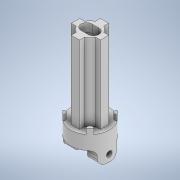
# Autodesk Inventor part: upper plug
Saved by Autodesk Inventor 2022 (Build 260153000, 153)
## iProperties
Created: 2022-03-20
Part Number: upper plug
Material: Generic
Document SubType Name: Modeling
Designer: Dahway
Density: 1 g/cm^3
Appearance: Default
Author: Dahway
Autodesk Inventor part; units mm, degrees
ref_plane "YZ Plane" through (0, 0, 0) normal (1, 0, 0) x (0, 1, 0)
ref_plane "XZ Plane" through (0, 0, 0) normal (0, 1, 0) x (-1, 0, 0)
ref_plane "XY Plane" through (0, 0, 0) normal (0, 0, 1) x (1, 0, 0)
sketch "Sketch1" plane through (0, 0, 0) normal (0, 1, 0) x (-1, 0, 0)
  circle A0 centre (0, 0) radius 7
  dimension "d0" = 14
  constraints: 1 centre point, 1 coincident
  measures "d0" diameter of A0
extrude "Extrusion1" add sketch "Sketch1" along normal blind 5
sketch "Sketch2" plane through (0, 5, 0) normal (0, 1, 0) x (1, 0, 0)
  circle A0 centre (0, 0) radius 3.75
  line L0 (-5.25, -1.5) -> (-2.25, -1.5)
  line L1 (-2.25, -1.5) -> (-2.25, 1.5)
  line L2 (-2.25, 1.5) -> (-5.25, 1.5)
  line L3 (-5.25, 1.5) -> (-5.25, -1.5)
  line L4 (-5.25, -1.5) -> (-2.25, 1.5) construction
  line L5 (-2.25, -1.5) -> (-5.25, 1.5) construction
  line L6 (-1.5, 2.25) -> (1.5, 2.25)
  line L7 (1.5, 2.25) -> (1.5, 5.25)
  line L8 (1.5, 5.25) -> (-1.5, 5.25)
  line L9 (-1.5, 5.25) -> (-1.5, 2.25)
  line L10 (-1.5, 2.25) -> (1.5, 5.25) construction
  line L11 (1.5, 2.25) -> (-1.5, 5.25) construction
  line L12 (2.25, -1.5) -> (5.25, -1.5)
  line L13 (5.25, -1.5) -> (5.25, 1.5)
  line L14 (5.25, 1.5) -> (2.25, 1.5)
  line L15 (2.25, 1.5) -> (2.25, -1.5)
  line L16 (2.25, -1.5) -> (5.25, 1.5) construction
  line L17 (5.25, -1.5) -> (2.25, 1.5) construction
  line L18 (-1.5, -5.25) -> (1.5, -5.25)
  line L19 (1.5, -5.25) -> (1.5, -2.25)
  line L20 (1.5, -2.25) -> (-1.5, -2.25)
  line L21 (-1.5, -2.25) -> (-1.5, -5.25)
  line L22 (-1.5, -5.25) -> (1.5, -2.25) construction
  line L23 (1.5, -5.25) -> (-1.5, -2.25) construction
  point P0 (-3.75, 0)
  point P1 (0, 3.75)
  point P2 (3.75, 0)
  point P3 (0, -3.75)
  point P4 (3.4369, 1.5)
  point P5 (1.5, 3.4369)
  point P6 (-1.5, 3.4369)
  point P7 (-3.4369, 1.5)
  point P8 (-3.4369, -1.5)
  point P9 (-1.5, -3.4369)
  point P10 (1.5, -3.4369)
  point P11 (3.4369, -1.5)
  dimension "d4" = 7.5
  dimension "d5" = 3
  dimension "d6" = 3
  dimension "d7" = 3
  dimension "d8" = 3
  dimension "d9" = 3
  dimension "d10" = 3
  dimension "d11" = 3
  dimension "d12" = 3
  constraints: 48 end point, 8 midpoint, 8 parallel, 4 horizontal, 4 perpendicular, 4 point on line, 3 point on circle, 1 centre point, 1 coincident
  measures "d4" diameter of A0
  measures "d5" distance of L2.end L1.end
  measures "d6" distance of L1.end L0.end
  measures "d7" distance of L8.end L7.end
  measures "d8" distance of L7.end L6.end
  measures "d9" distance of L14.end L13.end
  measures "d10" distance of L13.end L12.end
  measures "d11" distance of L20.end L19.end
  measures "d12" distance of L19.end L18.end
extrude "Extrusion2" add sketch "Sketch2" along normal blind 28
sketch "Sketch3" plane through (0, 33, 0) normal (0, 1, 0) x (1, 0, 0)
  circle A0 centre (-1.25, 0) radius 2
  circle A1 centre (1.25, 0) radius 2
  line L0 (-1.25, 2) -> (1.25, 2)
  line L1 (-1.0259, -1.9874) -> (1.4741, -1.9874)
  line L2 (-5.25, -1.5) -> (-3.4369, -1.5) projected
  line L3 (3.4369, -1.5) -> (5.25, -1.5) projected
  point P0 (0, 0)
  dimension "d15" = 4
  dimension "d16" = 4
  dimension "d19" = 2.5
  dimension "d21" = 1.25
  dimension "d22" = 1.5
  dimension "d23" = 1.5
  constraints: 4 end point, 4 point on circle, 2 centre point, 1 horizontal, 1 parallel, 1 tangent
  measures "d15" diameter of A0
  measures "d16" diameter of A1
  measures "d19" distance of A1.centre A0.centre
  measures "d21" distance of point (0, 0) A0.centre
  measures "d22" distance from line of L2 A0.centre
  measures "d23" distance from line of L3 A1.centre
extrude "Extrusion3" cut sketch "Sketch3" against normal blind 3 contours A0 A1 | L0 A1 A0 | A0 A1 L1 | A1 L1 A0 | A0 A1
sketch "Sketch4" plane through (0, 5, 0) normal (0, 1, 0) x (1, 0, 0)
  circle A0 centre (0, 0) radius 7 projected
  line L0 (0, 0) -> (7, 0) construction
  line L1 (0, 0) -> (7, 0) construction
  circle A1 centre (-4.9497, 4.9497) radius 1
  circle A2 centre (-4.9497, -4.9497) radius 1
  circle A3 centre (4.9497, -4.9497) radius 1
  circle A4 centre (4.9497, 4.9497) radius 1
  point P0 (-4.9497, -4.9497)
  point P1 (4.9497, 4.9497)
  point P2 (4.1939, 5.6045)
  point P3 (5.6045, 4.1939)
  point P4 (5.6045, -4.1939)
  point P5 (4.1939, -5.6045)
  point P6 (-5.6045, -4.1939)
  point P7 (-4.1939, -5.6045)
  point P8 (-4.1939, 5.6045)
  point P9 (-5.6045, 4.1939)
  dimension "d26" = 2
  dimension "d29" = 360
  constraints: 4 centre point, 4 end point, 2 horizontal, 2 point on circle, 1 coincident, 9 other
  measures "d26" diameter of A1
extrude "Extrusion4" add sketch "Sketch4" along normal blind 2 contours A4 A0 | A0 A3 | A1 A0 | A0 A2 picked at (4.7103, 4.7103) picked at (4.7103, -4.7103) picked at (-4.6879, 4.735) picked at (-4.6879, -4.735)
sketch "Sketch5" plane through (0, 0, 0) normal (0, -1, 0) x (1, 0, 0)
  line L0 (2.5, 3.45) -> (2.5, -3.45)
  arc A0 (5.6045, -4.1939) -> (5.6045, 4.1939) centre (0, 0) ccw projected
  arc A1 (6.0908, -3.45) -> (6.0908, 3.45) centre (0, 0) ccw
  line L1 (2.5, 3.45) -> (6.0908, 3.45)
  line L2 (2.5, -3.45) -> (6.0908, -3.45)
  dimension "d33" = 6.9
  dimension "d50" = 4.5
  constraints: 6 end point, 4 point on circle, 2 parallel, 1 centre point, 1 horizontal, 1 vertical
  measures "d33" distance of L0.start L0.end
  measures "d50" distance edge to line of A0 L0
extrude "Extrusion5" add sketch "Sketch5" along normal blind 5
pattern_circular "Circular Pattern1" count 2 over 360 about axis through (0, 0, 0) along (0, 1, 0) of "Extrusion5"
fillet "Fillet2" radius 2 10 edges at (4.2954, -5, -3.45) (4.2954, -5, 3.45) (-4.2954, -5, -3.45) (-4.2954, -5, 3.45) (4.2954, 0, -3.45) (-4.2954, 0, -3.45) (-4.2954, 0, 3.45) (4.2954, 0, 3.45) (2.5, 0, 0) (-2.5, 0, 0)
sketch "Sketch7" plane through (2.5, -3, -3.45) normal (-1, 0, 0) x (0, 0, 1)
  line L0 (4.9, -2) -> (2, -2) projected
  line L1 (0, 1) -> (0, 0) projected
  point P0 (3.45, 3)
  point P1 (3.45, 0.5)
  dimension "d52" = 2.5
  dimension "d53" = 3.45
  measures "d52" distance from line of L0 point (3.45, 0.5)
  measures "d53" distance from line of point (3.45, 0.5) L1
hole "Hole2" at (2.5, -2.5, 0) direction (1, 0, 0) diameter 2 end through all both
body "Solid1"
